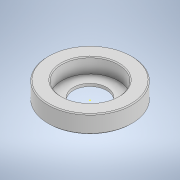
# Autodesk Inventor part: Bearing Spacer
Saved by Autodesk Inventor 2022 (Build 260153000, 153)
## iProperties
Created: 2021-09-20
Part Number: Bearing Spacer
Material: Generic
Document SubType Name: Modeling
Designer: LSabe
Density: 1 g/cm^3
Appearance: Default
Author: LSabe
Autodesk Inventor part; units mm, degrees
ref_plane "YZ Plane" through (0, 0, 0) normal (1, 0, 0) x (0, 1, 0)
ref_plane "XZ Plane" through (0, 0, 0) normal (0, 1, 0) x (-1, 0, 0)
ref_plane "XY Plane" through (0, 0, 0) normal (0, 0, 1) x (1, 0, 0)
sketch "Sketch1" plane through (0, 0, 0) normal (0, 1, 0) x (-1, 0, 0)
  point P0 (0, 0)
sketch "Sketch2" plane through (0, 0, 0) normal (0, 1, 0) x (-1, 0, 0)
  circle A0 centre (0, 0) radius 15.15
  circle A1 centre (0, 0) radius 17.65
  circle A2 centre (0, 0) radius 22.55
  circle A3 centre (0, 0) radius 20.05
  dimension "d0" = 30.3
  dimension "d1" = 2.5
  dimension "d2" = 45.1
  dimension "d3" = 2.5
  constraints: 4 centre point, 2 coincident
  measures "d0" diameter of A0
  measures "d1" radial gap between concentric circles of A0 A1
  measures "d2" diameter of A2
  measures "d3" radial gap between concentric circles of A2 A3
extrude "Extrusion1" add sketch "Sketch2" along normal blind 9.5 contours A1 | A2 | A3
sketch "Sketch3" plane through (0, 0, 0) normal (0, -1, 0) x (1, 0, 0)
  circle A0 centre (0, 0) radius 15.15 projected
  circle A1 centre (0, 0) radius 9
  dimension "d8" = 18
  constraints: 1 centre point, 1 coincident
  measures "d8" diameter of A1
extrude "Extrusion2" add sketch "Sketch3" against normal blind 1.5
chamfer "Chamfer1" distance 0.5 angle 45 3 edges at (22.55, 0, 0) (15.15, 9.5, 0) (22.55, 9.5, 0)
body "Solid1"
